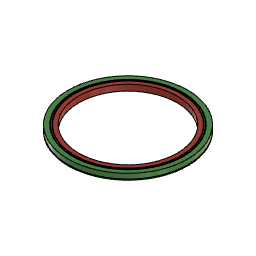
Cage (Autodesk Fusion 360 design; units mm, degrees)
Autodesk Fusion 360 part; units mm, degrees
sketch "Sketch1" plane through (0, 0, 0) normal (0, 0, 1) x (1, 0, 0)
  circle A0 centre (0, 0) radius 50
  circle A1 centre (0, 0) radius 54
  circle A2 centre (0, 0) radius 55 construction
  circle A3 centre (0, 0) radius 56
  circle A4 centre (0, 0) radius 60.5
  dimension "Gap_1" = 1
  dimension "d4_1" = 1
  dimension "bearingPCD_1" = 110
  dimension "pcdToID_1" = 5
  dimension "pcdToOD_1" = 5.5
  constraint coincident A0.centre A1.centre
  constraint concentric A2 A3
  constraint concentric A0 A4
  measures "Gap_1" distance of A1 A2
  measures "d4_1" distance of A2 A3
  measures "bearingPCD_1" diameter of A2
  measures "pcdToID_1" distance of A0 A2
  measures "pcdToOD_1" distance of A2 A4
sketch "Sketch2" plane through (0, 0, 0) normal (0, 1, 0) x (1, 0, 0)
  line L0 (-55, 0) -> (55, 0)
  line L1 (55, 0) -> (55, -3) construction
  circle A0 centre (55, -3) radius 2.25
  dimension "d9_1" = 3
  dimension "d10_1" = 4.5
  constraint coincident L0.end L1.start
  constraint perpendicular L0 L1
  constraint coincident L1.end A0.centre
  measures "d9_1" distance of L0.end L1.end
  measures "d10_1" diameter of A0
extrude "Extrude1" add sketch "Sketch1" along normal blind 6 makes body 1 at (53.9329, -2.6917, 4) makes body 2 at (60.4248, -3.0157, 4)
revolve "Revolve1" cut sketch "Sketch2" angle 360 about axis through (0, 0, 1.75) along (0, 0, 1) bodies 1 2
ref_plane "WorkPlane1" through (0, 0, 3) normal (0, 0, 1) x (1, 0, 0)
split "Split1" by plane through (0, 0, 3) normal (0, 0, 1) bodies 2 makes body 3 at (58.5663, -5.7878, 6)
sketch "Sketch3" plane through (0, 0, 3) normal (0, 0, 1) x (-1, 0, 0)
  circle A0 centre (0, 0) radius 57.25
  circle A1 centre (0, 0) radius 60.5
  circle A2 centre (0, 0) radius 59.25
  dimension "d13_1" = 118.5
  constraint coincident A0.centre A1.centre
  measures "d13_1" diameter of A2
extrude "Extrude2" cut sketch "Sketch3" against normal blind 2 contours A1 bodies 2
extrude "Extrude3" add sketch "Sketch3" against normal blind 2 contours A1 bodies 3
sketch "Sketch4" plane through (0, 0, 0) normal (0, 0, 1) x (1, 0, 0)
  circle A0 centre (0, 0) radius 55 construction
  circle A1 centre (0, 0) radius 54.5
  circle A2 centre (0, 0) radius 55.5
  dimension "cageWidth" = 1
  dimension "d26" = 0.5
  constraint concentric A0 A1
  constraint concentric A1 A2
  measures "cageWidth" distance of A1 A2
  measures "d26" distance of A0 A2
extrude "Extrude4" add sketch "Sketch4" along normal blind 6 separate body makes body 4
sketch "Sketch5" plane through (0, 0, 0) normal (1, 0, 0) x (0, 1, 0)
  line L0 (0, 0) -> (0, 3) construction
  circle A0 centre (0, 3) radius 2.25 construction
  circle A1 centre (0, 3) radius 2.45
  dimension "d29" = 3
  dimension "d30" = 4.5
  dimension "cageClearance" = 0.2
  constraint coincident L0.start origin
  constraint vertical L0
  constraint coincident L0.end A0.centre
  constraint concentric A0 A1
  measures "d29" distance of L0.start L0.end
  measures "d30" diameter of A0
  measures "cageClearance" distance of A0 A1
extrude "Extrude5" cut sketch "Sketch5" along normal through all bodies 4
pattern_circular "C-Pattern1" count 40 over 360 about axis through (0, 0, 1.75) along (0, 0, 1) of "Extrude5"
move_face "OffsetFaces1" offset -0.1 1 faces at (58.9556, -5.8994, 2.3333) on bodies 2
move_face "OffsetFaces2" offset -0.2 1 faces at (-58.0833, 5.7828, 3) on bodies 2
equation "d4_1 = Gap_1"
equation "d7_1 = height"
equation "d9_1 = height / 2"
equation "d12_1 = height / 2"
equation "d13_1 = pcdToOD_1 + bearingPCD_1 + 3 mm"
equation "d26 = cageWidth / 2"
equation "d27 = height"
equation "d29 = height / 2"
equation "d30 = balldiameter"
equation "numOfBalls = 40"
equation "height = 6 mm"
equation "balldiameter = 4.5 mm"
